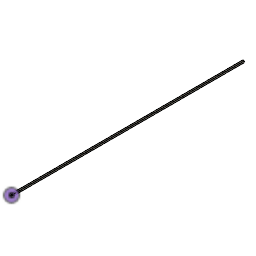
A3 (Autodesk Fusion 360 design; units mm, degrees)
part number: 2026-09-03-16-34-26-926
Autodesk Fusion 360 part; units mm, degrees
sketch "Sketch4" plane through (0, 0, 0) normal (0, 1, 0) x (1, 0, 0)
  line L0 (0, 0) -> (12.7, 0)
  line L1 (12.7, 0) -> (12.7, -12.7)
  line L2 (12.7, -12.7) -> (0, -12.7)
  line L3 (0, -12.7) -> (0, 0)
  dimension "d19" = 12.7
  constraint horizontal L0
  constraint vertical L1
  constraint horizontal L2
  constraint vertical L3
  constraint coincident L0.start L3.end
  constraint equal L0 L3
  measures "d19" distance of L0.start L2.end
extrude "Extrude4" add sketch "Sketch4" along normal blind 33.02 makes body 1
delete_body "RemoveBody1" bodies 1
extrude "Extrude5" add sketch "Sketch4" along normal blind 1905 separate body makes body 2
equation "Force = 300 lbforce"
equation "Elastic_modulus = 10000000 psi"
equation "Deflection = 0.009 in"
equation "Side = 0.5 in"
equation "Length = Deflection * Side ^ 2 * Elastic_modulus / Force"
equation "d19 = Side"
equation "d22 = Length"
